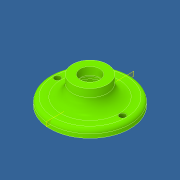
# Autodesk Inventor part: Wrist_Cover_2
Saved by Autodesk Inventor 2016 (Build 200138000, 138)
## iProperties
Created: 2015-09-10
Part Number: Wrist_Cover_2
Material: ABS-Kunststoff
Document SubType Name: Modeling
Designer: 4ndreas
Density: 1.06 g/cm^3
Appearance: Glatt - grün
Mass: 5.28366 g
Surface Area: 37.8444 cm^2
Volume: 4.98458 cm^3
Author: 4ndreas
Autodesk Inventor part; units mm, degrees
ref_plane "YZ Plane" through (0, 0, 0) normal (1, 0, 0) x (0, 1, 0)
ref_plane "XZ Plane" through (0, 0, 0) normal (0, 1, 0) x (-1, 0, 0)
ref_plane "XY Plane" through (0, 0, 0) normal (0, 0, 1) x (1, 0, 0)
sketch "Skizze1" plane through (0, 0, 0) normal (0, 0, 1) x (1, 0, 0)
  circle A0 centre (16.76, 0) radius 1.25 projected
  circle A1 centre (-16.76, 0) radius 1.25 projected
  line L0 (-6.25, 16) -> (-11.9414, 16) projected
  line L1 (-2.25, 20) -> (-6.25, 16) projected
  line L2 (2.25, 20) -> (-2.25, 20) projected
  line L3 (6.25, 16) -> (2.25, 20) projected
  line L4 (11.9414, 16) -> (6.25, 16) projected
  line L5 (11.9414, 16) -> (12.9414, 15) projected
  line L6 (12.9414, -15) -> (12.9414, 15) projected
  line L7 (11.9414, -16) -> (12.9414, -15) projected
  line L8 (-11.9414, -16) -> (11.9414, -16) projected
  line L9 (-11.9414, -16) -> (-12.9414, -15) projected
  line L10 (-12.9414, 15) -> (-12.9414, -15) projected
  line L11 (-12.9414, 15) -> (-11.9414, 16) projected
  circle A2 centre (0, 0) radius 20.5786 projected
  point P0 (0, 0)
extrude "Extrusion1" add sketch "Skizze1" along normal blind 4 contours L1 L2 L3 L4 L5 L6 L7 L8 L9 L10 L11 L0 | A2
sketch "Skizze2" plane through (0, 0, 4) normal (0, 0, 1) x (1, 0, 0)
  point P0 (0, 0)
sketch "Skizze3" plane through (0, 0, 4) normal (0, 0, 1) x (1, 0, 0)
  line L0 (-12.1, -11.9394) -> (-9.9, -11.9394)
  line L1 (-9.9, -11.9394) -> (-9.9, 11.9394)
  line L2 (-9.9, 11.9394) -> (-12.1, 11.9394)
  line L3 (-12.1, 11.9394) -> (-12.1, -11.9394)
  line L4 (-7.7, 14.502) -> (-5.5, 14.502)
  line L5 (-5.5, 14.502) -> (-5.5, -14.502)
  line L6 (-5.5, -14.502) -> (-7.7, -14.502)
  line L7 (-7.7, -14.502) -> (-7.7, 14.502)
  line L8 (-3.3, 15.4709) -> (-1.1, 15.4709)
  line L9 (-1.1, 15.4709) -> (-1.1, -15.4709)
  line L10 (-1.1, -15.4709) -> (-3.3, -15.4709)
  line L11 (-3.3, -15.4709) -> (-3.3, 15.4709)
  circle A0 centre (-16.76, 0) radius 1.25 projected
  circle A1 centre (16.76, 0) radius 1.25 projected
  circle A2 centre (0, 0) radius 20.5786 projected
  line L12 (-16.76, 0) -> (0, 0) construction
  circle A3 centre (0, 0) radius 15.51 construction
  line L13 (0, 0) -> (0, 15.51)
  point P0 (0, 0)
  dimension "d2" = 2.2
  dimension "d3" = 2.2
  dimension "d4" = 2.2
  dimension "d5" = 2.2
  dimension "d6" = 2.2
  dimension "d7" = 1.1
  constraints: 28 end point, 6 parallel, 4 horizontal, 3 perpendicular, 1 coincident, 1 vertical, 10 other
  measures "d2" distance between parallel lines of L11 L9
  measures "d3" distance between parallel lines of L7 L5
  measures "d4" distance between parallel lines of L3 L1
  measures "d5" distance between parallel lines of L1 L7
  measures "d6" distance between parallel lines of L5 L11
  measures "d7" distance from line of L9 L12.end
ref_plane "Arbeitsebene1" through (0, 0, 4) normal (1, 0, 0) x (0, 1, 0)
extrude "Extrusion2" cut sketch "Skizze3" against normal through all contours L3 L2 L1 L0 | L4 L5 L6 L7 | L8 L9 L10 L11
mirror "Spiegeln1" about plane through (0, 0, 4) normal (1, 0, 0) of "Extrusion2"
sketch "Skizze4" plane through (0, 0, 4) normal (0, 0, 1) x (1, 0, 0)
  line L0 (5.5, -14.502) -> (5.5, 14.502) projected
  line L1 (5.5, 14.502) -> (7.7, 14.502) projected
  line L2 (7.7, 14.502) -> (7.7, -14.502) projected
  line L3 (7.7, -14.502) -> (5.5, -14.502) projected
  line L4 (1.1, -15.4709) -> (1.1, 15.4709) projected
  line L5 (1.1, 15.4709) -> (3.3, 15.4709) projected
  line L6 (3.3, 15.4709) -> (3.3, -15.4709) projected
  line L7 (3.3, -15.4709) -> (1.1, -15.4709) projected
  line L8 (9.9, 11.9394) -> (12.1, 11.9394) projected
  line L9 (12.1, 11.9394) -> (12.1, -11.9394) projected
  line L10 (12.1, -11.9394) -> (9.9, -11.9394) projected
  line L11 (9.9, -11.9394) -> (9.9, 11.9394) projected
  line L12 (-7.7, -14.502) -> (-7.7, 14.502) projected
  line L13 (-7.7, 14.502) -> (-5.5, 14.502) projected
  line L14 (-5.5, 14.502) -> (-5.5, -14.502) projected
  line L15 (-5.5, -14.502) -> (-7.7, -14.502) projected
  line L16 (-9.9, 11.9394) -> (-9.9, -11.9394) projected
  line L17 (-9.9, -11.9394) -> (-12.1, -11.9394) projected
  line L18 (-12.1, -11.9394) -> (-12.1, 11.9394) projected
  line L19 (-12.1, 11.9394) -> (-9.9, 11.9394) projected
  line L20 (-3.3, -15.4709) -> (-3.3, 15.4709) projected
  line L21 (-3.3, 15.4709) -> (-1.1, 15.4709) projected
  line L22 (-1.1, 15.4709) -> (-1.1, -15.4709) projected
  line L23 (-1.1, -15.4709) -> (-3.3, -15.4709) projected
  circle A0 centre (-16.76, 0) radius 1.25 projected
  circle A1 centre (16.76, 0) radius 1.25 projected
  circle A2 centre (0, 0) radius 20.5786 projected
  point P0 (0, 0)
hole "Bohrung1" at (-16.76, 0, 4) at (16.76, 0, 4) direction (0, 0, -1) diameter 3.2 end through all
sketch "Skizze5" plane through (0, 0, 4) normal (0, 0, 1) x (1, 0, 0)
  circle A0 centre (-16.76, 0) radius 1.6 projected
  circle A1 centre (16.76, 0) radius 1.6 projected
  line L0 (5.5, -14.502) -> (5.5, 14.502) projected
  line L1 (5.5, 14.502) -> (7.7, 14.502) projected
  line L2 (7.7, 14.502) -> (7.7, -14.502) projected
  line L3 (7.7, -14.502) -> (5.5, -14.502) projected
  line L4 (1.1, -15.4709) -> (1.1, 15.4709) projected
  line L5 (1.1, 15.4709) -> (3.3, 15.4709) projected
  line L6 (3.3, 15.4709) -> (3.3, -15.4709) projected
  line L7 (3.3, -15.4709) -> (1.1, -15.4709) projected
  line L8 (9.9, 11.9394) -> (12.1, 11.9394) projected
  line L9 (12.1, 11.9394) -> (12.1, -11.9394) projected
  line L10 (12.1, -11.9394) -> (9.9, -11.9394) projected
  line L11 (9.9, -11.9394) -> (9.9, 11.9394) projected
  line L12 (-7.7, -14.502) -> (-7.7, 14.502) projected
  line L13 (-7.7, 14.502) -> (-5.5, 14.502) projected
  line L14 (-5.5, 14.502) -> (-5.5, -14.502) projected
  line L15 (-5.5, -14.502) -> (-7.7, -14.502) projected
  line L16 (-9.9, 11.9394) -> (-9.9, -11.9394) projected
  line L17 (-9.9, -11.9394) -> (-12.1, -11.9394) projected
  line L18 (-12.1, -11.9394) -> (-12.1, 11.9394) projected
  line L19 (-12.1, 11.9394) -> (-9.9, 11.9394) projected
  line L20 (-3.3, -15.4709) -> (-3.3, 15.4709) projected
  line L21 (-3.3, 15.4709) -> (-1.1, 15.4709) projected
  line L22 (-1.1, 15.4709) -> (-1.1, -15.4709) projected
  line L23 (-1.1, -15.4709) -> (-3.3, -15.4709) projected
  circle A2 centre (0, 0) radius 20.5786 projected
  point P0 (0, 0)
extrude "Extrusion3" add sketch "Skizze5" against normal up to surface (4 mm away) contours L0 L1 L2 L3 | L4 L5 L6 L7 | L8 L9 L10 L11 | L12 L13 L14 L15 | L16 L17 L18 L19 | L20 L21 L22 L23
sketch "Skizze6" plane through (0, 0, 4) normal (0, 0, 1) x (1, 0, 0)
  circle A0 centre (0, 0) radius 9
  circle A1 centre (0, 0) radius 7
  dimension "d20" = 18
  dimension "d21" = 2
  constraints: 2 centre point, 2 coincident
  measures "d20" diameter of A0
  measures "d21" radial gap between concentric circles of A0 A1
extrude "Extrusion4" add sketch "Skizze6" along normal blind 10
sketch "Skizze9" plane through (0, 0, 4) normal (0, 0, 1) x (1, 0, 0)
  circle A0 centre (0, 0) radius 7 projected
extrude "Extrusion6" cut sketch "Skizze9" against normal through all
sketch "Skizze10" plane through (0, 0, 14) normal (0, 0, 1) x (1, 0, 0)
  circle A0 centre (0, 0) radius 7 projected
  circle A1 centre (0, 0) radius 9 projected
  circle A2 centre (0, 0) radius 5
  dimension "d28" = 10
  constraints: 1 centre point, 1 coincident
  measures "d28" diameter of A2
extrude "Extrusion7" add sketch "Skizze10" against normal blind 4 contours A0
chamfer "Fase1" distance 2 angle 45 1 edges at (-7, 0, 10)
fillet "Rundung1" radius 6 1 edges at (-9, 0, 4)
sketch "Skizze11" plane through (0, 0, 0) normal (0, 0, -1) x (-1, 0, 0)
  point P0 (0, 0)
chamfer "Fase2" distance 7 angle 45 1 edges at (-7, 0, 0)
fillet "Rundung2" radius 2 1 edges at (-20.5786, 0, 4)
sketch "Skizze7" plane through (0, 0, 14) normal (0, 0, 1) x (1, 0, 0)
  circle A0 centre (0, 0) radius 7 projected
equation "\"d3\" = d2"
equation "\"d4\" = d3"
equation "\"d5\" = d4"
equation "\"d6\" = d3"
equation "\"d7\" = 0.5 * d2"
